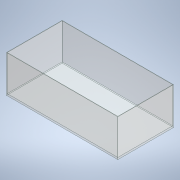
# Autodesk Inventor part: Tank
Saved by Autodesk Inventor 2020.2 (Build 242310000, 310)
## iProperties
Created: 2019-12-22
Part Number: Tank
Material: Glass
Document SubType Name: Modeling
Designer: Andrew
Density: 2.18 g/cm^3
Appearance: Clear
Author: Andrew
Autodesk Inventor part; units mm, degrees
ref_plane "YZ Plane" through (0, 0, 0) normal (1, 0, 0) x (0, 1, 0)
ref_plane "XZ Plane" through (0, 0, 0) normal (0, 1, 0) x (-1, 0, 0)
ref_plane "XY Plane" through (0, 0, 0) normal (0, 0, 1) x (1, 0, 0)
sketch "Sketch2" plane through (0, 0, 0) normal (0, 1, 0) x (-1, 0, 0)
  line L0 (457.2, 228.6) -> (-457.2, 228.6)
  line L1 (-457.2, 228.6) -> (-457.2, -228.6)
  line L2 (-457.2, -228.6) -> (457.2, -228.6)
  line L3 (457.2, -228.6) -> (457.2, 228.6)
  line L4 (457.2, 228.6) -> (-457.2, -228.6) construction
  line L5 (-457.2, 228.6) -> (457.2, -228.6) construction
  line L6 (454.025, 225.425) -> (-454.025, 225.425)
  line L7 (-454.025, 225.425) -> (-454.025, -225.425)
  line L8 (-454.025, -225.425) -> (454.025, -225.425)
  line L9 (454.025, -225.425) -> (454.025, 225.425)
  line L10 (454.025, 225.425) -> (-454.025, -225.425) construction
  line L11 (-454.025, 225.425) -> (454.025, -225.425) construction
  point P0 (0, 0)
  dimension "d0" = 914.4
  dimension "d1" = 457.2
  dimension "d2" = 3.175
  dimension "d3" = 3.175
  constraints: 24 end point, 4 midpoint, 4 parallel, 2 horizontal, 2 perpendicular
  measures "d0" distance of L0.start L0.end
  measures "d1" distance of L0.end L1.end
  measures "d2" distance between parallel lines of L2 L8
  measures "d3" distance between parallel lines of L7 L1
extrude "Extrusion1" add sketch "Sketch2" along normal blind 304.8
extrude "Extrusion2" add sketch "Sketch2" along normal blind 12.7 contours L3 L2 L1 L0 | L9 L8 L7 L6
body "Solid1"
